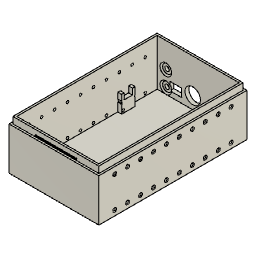
Outer Case Bottom v69 (Autodesk Fusion 360 design; units mm, degrees)
Autodesk Fusion 360 part; units mm, degrees
sketch "Sketch1" plane through (0, 0, 0) normal (0, 0, 1) x (1, 0, 0)
  line L0 (0, 0) -> (0, 12)
  line L1 (0, 12) -> (-3, 12)
  line L2 (-3, 12) -> (-3, 17)
  line L3 (-3, 17) -> (0, 17)
  line L4 (0, 17) -> (0, 79)
  line L5 (0, 79) -> (-3, 79)
  line L6 (-3, 79) -> (-3, 84)
  line L7 (-3, 84) -> (0, 84)
  line L8 (0, 84) -> (0, 96)
  line L9 (0, 96) -> (56, 96)
  line L10 (56, 96) -> (56, 84)
  line L11 (56, 84) -> (59, 84)
  line L12 (59, 84) -> (59, 79)
  line L13 (59, 79) -> (56, 79)
  line L14 (56, 79) -> (56, 17)
  line L15 (56, 17) -> (59, 17)
  line L16 (59, 17) -> (59, 12)
  line L17 (59, 12) -> (56, 12)
  line L18 (56, 12) -> (56, 0)
  line L19 (56, 0) -> (0, 0)
  line L20 (-0.7, -0.7) -> (-0.7, 11.3)
  line L21 (-0.7, 11.3) -> (-3.7, 11.3)
  line L22 (-3.7, 11.3) -> (-3.7, 17.7)
  line L23 (-3.7, 17.7) -> (-0.7, 17.7)
  line L24 (-0.7, 17.7) -> (-0.7, 78.3)
  line L25 (-0.7, 78.3) -> (-3.7, 78.3)
  line L26 (-3.7, 78.3) -> (-3.7, 84.7)
  line L27 (-3.7, 84.7) -> (-0.7, 84.7)
  line L28 (-0.7, 84.7) -> (-0.7, 96.7)
  line L29 (-0.7, 96.7) -> (56.7, 96.7)
  line L30 (56.7, 96.7) -> (56.7, 84.7)
  line L31 (56.7, 84.7) -> (59.7, 84.7)
  line L32 (59.7, 84.7) -> (59.7, 78.3)
  line L33 (59.7, 78.3) -> (56.7, 78.3)
  line L34 (56.7, 78.3) -> (56.7, 17.7)
  line L35 (56.7, 17.7) -> (59.7, 17.7)
  line L36 (59.7, 17.7) -> (59.7, 11.3)
  line L37 (59.7, 11.3) -> (56.7, 11.3)
  line L38 (56.7, 11.3) -> (56.7, -0.7)
  line L39 (56.7, -0.7) -> (-0.7, -0.7)
  line L40 (-3.7, 106.7) -> (59.7, 106.7)
  line L41 (59.7, 106.7) -> (59.7, -1.7)
  line L42 (59.7, -1.7) -> (-3.7, -1.7)
  line L43 (-3.7, -1.7) -> (-3.7, 106.7)
  line L44 (62.7, -4.7) -> (-6.7, -4.7)
  line L45 (-6.7, -4.7) -> (-6.7, 109.7)
  line L46 (-6.7, 109.7) -> (62.7, 109.7)
  line L47 (62.7, 109.7) -> (62.7, -4.7)
  line L48 (-3.7, 86.7) -> (-0.7, 86.7)
  line L49 (-0.7, 86.7) -> (-0.7, 76.3)
  line L50 (-0.7, 76.3) -> (-3.7, 76.3)
  line L51 (-3.7, 76.3) -> (-3.7, 86.7)
  line L52 (-3.7, 19.7) -> (-0.7, 19.7)
  line L53 (-0.7, 19.7) -> (-0.7, 9.3)
  line L54 (-0.7, 9.3) -> (-3.7, 9.3)
  line L55 (-3.7, 9.3) -> (-3.7, 19.7)
  line L56 (59.7, 19.7) -> (56.7, 19.7)
  line L57 (56.7, 19.7) -> (56.7, 9.3)
  line L58 (56.7, 9.3) -> (59.7, 9.3)
  line L59 (59.7, 9.3) -> (59.7, 19.7)
  line L60 (59.7, 86.7) -> (56.7, 86.7)
  line L61 (56.7, 86.7) -> (56.7, 76.3)
  line L62 (56.7, 76.3) -> (59.7, 76.3)
  line L63 (59.7, 76.3) -> (59.7, 86.7)
  dimension "d1" = 56
  dimension "d2" = 5
  dimension "d3" = 12
  dimension "d4" = 5
  dimension "d5" = 12
  dimension "d6" = 3
  dimension "d7" = 3
  dimension "d8" = -0.7
  dimension "d9" = -3
  dimension "d10" = 10
  dimension "d11" = 1
  dimension "d12" = 2
  dimension "d13" = 2
  dimension "d14" = 2
  dimension "d15" = 2
  dimension "d16" = 2
  dimension "d17" = 2
  dimension "d18" = 2
  dimension "d19" = 2
  dimension "d28" = 96
  constraint coincident L0.start L19.end
  constraint vertical L0
  constraint perpendicular L0 L1
  constraint perpendicular L1 L2
  constraint perpendicular L2 L3
  constraint perpendicular L3 L4
  constraint perpendicular L2 L5
  constraint perpendicular L5 L6
  constraint perpendicular L2 L7
  constraint perpendicular L7 L8
  constraint perpendicular L8 L9
  constraint perpendicular L9 L10
  constraint perpendicular L8 L11
  constraint perpendicular L11 L12
  constraint perpendicular L12 L13
  constraint perpendicular L13 L14
  constraint perpendicular L14 L15
  constraint perpendicular L15 L16
  constraint perpendicular L16 L17
  constraint perpendicular L17 L18
  constraint perpendicular L0 L19
  constraint collinear L4 L8
  constraint collinear L0 L4
  constraint collinear L10 L14
  constraint horizontal L6.end L11.end
  constraint horizontal L5.end L12.end
  constraint horizontal L2.end L15.end
  constraint horizontal L1.end L16.end
  constraint vertical L2.end L6.end
  constraint vertical L11.end L15.end
  constraint horizontal L40
  constraint vertical L41
  constraint horizontal L42
  constraint vertical L43
  constraint horizontal L48
  constraint vertical L49
  constraint horizontal L50
  constraint vertical L51
  constraint coincident L24 L49.end
  constraint coincident L43 L48.start
  constraint horizontal L52
  constraint vertical L53
  constraint horizontal L54
  constraint vertical L55
  constraint coincident L20 L53.end
  constraint coincident L43 L52.start
  constraint horizontal L56
  constraint vertical L57
  constraint horizontal L58
  constraint vertical L59
  constraint coincident L38 L57.end
  constraint coincident L41 L56.start
  constraint horizontal L60
  constraint vertical L61
  constraint horizontal L62
  constraint vertical L63
  constraint coincident L34 L61.end
  constraint coincident L41 L60.start
  constraint vertical L14.end L17.end
  measures "d1" distance of L8.end L9.end
  measures "d2" distance of L5.end L6.end
  measures "d3" distance of L7 L9
  measures "d4" distance of L1.end L2.end
  measures "d5" distance of L1 L19
  measures "d6" distance of L6.end L7.end
  measures "d7" distance of L10.end L11.end
  measures "d10" distance of L29 L40
  measures "d11" distance of L39 L42
  measures "d12" distance of L27 L48
  measures "d13" distance of L25 L50
  measures "d14" distance of L23 L52
  measures "d15" distance of L21 L54
  measures "d16" distance of L35 L56
  measures "d17" distance of L37 L58
  measures "d18" distance of L31 L60
  measures "d19" distance of L33 L62
  measures "d28" distance of L9 L19
extrude "Extrude4" add sketch "Sketch1" along normal blind 10.6 contours L1 L2 L3 L21 L22 L23 L43 L53 L55 | L1 L2 L3 L53 | L15 L16 L17 L57 | L15 L16 L17 L35 L36 L37 L41 L57 L59 | L5 L6 L7 L25 L26 L27 L43 L49 L51 | L5 L6 L7 L49 | L11 L12 L13 L61 | L11 L12 L13 L31 L32 L33 L41 L61 L63 makes body 1 at (56.7, 82.5667, 3.5333) makes body 2 at (59.7, 13.4333, 7.0667) makes body 3 at (-0.7, 82.5667, 3.5333) makes body 4 at (-0.7, 15.5667, 3.5333)
extrude "Extrude3" add sketch "Sketch1" along normal blind 15.2 contours L20 L21 L43 L53 L54 L55 | L23 L24 L43 L52 L53 L55 | L37 L38 L41 L57 L58 L59 | L34 L35 L41 L56 L57 L59 | L24 L25 L43 L49 L50 L51 | L33 L34 L41 L61 L62 L63 | L27 L28 L43 L48 L49 L51 | L30 L31 L41 L60 L61 L63 bodies 1 2 3 4
extrude "Extrude2" add sketch "Sketch1" along normal blind 33 bodies 1 2 3 4
extrude "Extrude1" add sketch "Sketch1" along normal blind 2 contours L0 L1 L17 L18 L19 L20 L38 L39 L53 L57 | L0 L1 L3 L4 L5 L7 L8 L9 L10 L11 L13 L14 L15 L17 L18 L19 L49 L53 L57 L61 | L1 L2 L3 L21 L22 L23 L43 L53 L55 | L1 L2 L3 L53 | L3 L4 L5 L24 L49 L53 | L20 L21 L43 L53 L54 L55 | L15 L16 L17 L57 | L15 L16 L17 L35 L36 L37 L41 L57 L59 | L23 L24 L43 L52 L53 L55 | L20 L38 L39 L41 L42 L43 L54 L58 | L13 L14 L15 L34 L57 L61 | L37 L38 L41 L57 L58 L59 | L24 L43 L50 L52 | L34 L35 L41 L56 L57 L59 | L5 L6 L7 L25 L26 L27 L43 L49 L51 | L5 L6 L7 L49 | L24 L25 L43 L49 L50 L51 | L34 L41 L56 L62 | L7 L8 L9 L10 L11 L28 L29 L30 L49 L61 | L11 L12 L13 L61 | L11 L12 L13 L31 L32 L33 L41 L61 L63 | L33 L34 L41 L61 L62 L63 | L27 L28 L43 L48 L49 L51 | L28 L29 L30 L40 L41 L43 L48 L60 | L30 L31 L41 L60 L61 L63 | L44 L45 L46 L47 bodies 1
sketch "Sketch2" plane through (0, 0, 33) normal (0, 0, 1) x (-1, 0, 0)
  line L0 (-62.7, -109.7) -> (6.7, -109.7)
  line L1 (6.7, -109.7) -> (6.7, 4.7)
  line L2 (6.7, 4.7) -> (-62.7, 4.7)
  line L3 (-62.7, 4.7) -> (-62.7, -109.7)
  line L4 (-59.7, -106.7) -> (-59.7, 1.7)
  line L5 (-59.7, 1.7) -> (3.7, 1.7)
  line L6 (3.7, 1.7) -> (3.7, -106.7)
  line L7 (3.7, -106.7) -> (-59.7, -106.7)
  line L8 (-61.2, 3.2) -> (-61.2, -108.2)
  line L9 (-61.2, -108.2) -> (5.2, -108.2)
  line L10 (5.2, -108.2) -> (5.2, 3.2)
  line L11 (5.2, 3.2) -> (-61.2, 3.2)
  line L12 (3.7, -117.1) -> (3.7, -106.7)
  line L13 (-59.7, -19.7) -> (-59.7, -9.3)
  line L14 (3.7, -86.7) -> (3.7, -76.3)
  line L15 (-59.7, -86.7) -> (-59.7, -76.3)
  dimension "d29" = -1.5
  constraint coincident L6.end L7.start
extrude "Extrude5" add sketch "Sketch2" along normal blind 5 contours L8 L9 L10 L11 bodies 1
sketch "Sketch3" plane through (0, 106.7, 0) normal (0, -1, 0) x (1, 0, 0)
  line L0 (-3.7, 2) -> (59.7, 2)
  line L1 (59.7, 2) -> (59.7, 38)
  line L2 (59.7, 38) -> (-3.7, 38)
  line L3 (-3.7, 38) -> (-3.7, 2)
  circle A0 centre (53, 6.5) radius 1.7
  circle A1 centre (3, 6.5) radius 1.7
  circle A2 centre (53, 18.5) radius 1.7
  circle A3 centre (3, 18.5) radius 1.7
  line L4 (36, 12.3) -> (47.3, 12.3)
  line L5 (47.3, 12.3) -> (47.3, 6.4)
  line L6 (47.3, 6.4) -> (36, 6.4)
  line L7 (36, 6.4) -> (36, 12.3)
  line L8 (6.2, 5.9) -> (15.1, 5.9)
  line L9 (15.1, 5.9) -> (15.1, 12.2)
  line L10 (15.1, 12.2) -> (6.2, 12.2)
  line L11 (6.2, 12.2) -> (6.2, 5.9)
  line L12 (36, 12.3) -> (33, 12.3)
  line L13 (33, 12.3) -> (33, 14.3)
  line L14 (33, 14.3) -> (36, 14.3)
  line L15 (36, 14.3) -> (36, 12.3)
  line L16 (36, 6.4) -> (33, 6.4)
  line L17 (33, 6.4) -> (33, 4.4)
  line L18 (33, 4.4) -> (36, 4.4)
  line L19 (36, 4.4) -> (36, 6.4)
  line L20 (47.3, 12.3) -> (50.3, 12.3)
  line L21 (50.3, 12.3) -> (50.3, 14.3)
  line L22 (50.3, 14.3) -> (47.3, 14.3)
  line L23 (47.3, 14.3) -> (47.3, 12.3)
  line L24 (47.3, 6.4) -> (50.3, 6.4)
  line L25 (50.3, 6.4) -> (50.3, 4.4)
  line L26 (50.3, 4.4) -> (47.3, 4.4)
  line L27 (47.3, 4.4) -> (47.3, 6.4)
  circle A4 centre (3, 18.5) radius 3.5
  circle A5 centre (3, 6.5) radius 3.5
  circle A6 centre (53, 18.5) radius 3.5
  circle A7 centre (53, 6.5) radius 3.5
  dimension "d32" = 3.4
  dimension "d35" = -50
  dimension "d36" = 12
  dimension "d37" = 4.5
  dimension "d38" = 6.7
  dimension "d41" = 50
  dimension "d42" = 63.4
  dimension "d43" = 12.4
  dimension "d45" = 5.9
  dimension "d46" = 11.3
  dimension "d47" = 8.9
  dimension "d48" = 6.3
  dimension "d49" = 3.9
  dimension "d51" = 3
  dimension "d52" = 2
  dimension "d53" = 3
  dimension "d54" = 2
  dimension "d55" = 3
  dimension "d56" = 2
  dimension "d57" = 3
  dimension "d58" = 2
  dimension "d74" = 4.4
  dimension "d75" = 7
  dimension "d76" = 7
  dimension "d77" = 7
  dimension "d78" = 7
  dimension "d113" = 9.9
  constraint horizontal L4
  constraint vertical L5
  constraint horizontal L6
  constraint vertical L7
  constraint horizontal L8
  constraint vertical L9
  constraint horizontal L10
  constraint vertical L11
  constraint horizontal L12
  constraint vertical L13
  constraint horizontal L14
  constraint vertical L15
  constraint horizontal L16
  constraint vertical L17
  constraint horizontal L18
  constraint vertical L19
  constraint horizontal L20
  constraint vertical L21
  constraint horizontal L22
  constraint vertical L23
  constraint horizontal L24
  constraint vertical L25
  constraint horizontal L26
  constraint vertical L27
  constraint concentric A3 A4
  constraint concentric A1 A5
  constraint concentric A2 A6
  constraint concentric A0 A7
  measures "d32" diameter of A0
  measures "d37" distance of L0 A0.centre
  measures "d38" distance of L1 A0.centre
  measures "d41" distance of A2.centre A3.centre
  measures "d42" distance of L1.end L2.end
  measures "d43" distance of L1 L5
  measures "d45" distance of L4.start L6.end
  measures "d46" distance of L4.start L4.end
  measures "d47" distance of L8.start L8.end
  measures "d48" distance of L8.start L10.end
  measures "d49" distance of L0 L8
  measures "d51" distance of L4.start L12.end
  measures "d52" distance of L4.start L14.end
  measures "d53" distance of L6.end L16.end
  measures "d54" distance of L6.end L18.end
  measures "d55" distance of L4.end L20.end
  measures "d56" distance of L4.end L22.end
  measures "d57" distance of L5.end L24.end
  measures "d58" distance of L5.end L26.end
  measures "d74" distance of L0 L6
  measures "d75" diameter of A4
  measures "d76" diameter of A5
  measures "d77" diameter of A6
  measures "d78" diameter of A7
  measures "d113" distance of L3 L11
extrude "Extrude9" cut sketch "Sketch3" against normal blind 1 contours L24 L25 L26 A7 | L24 L25 L26 A7 | L8 L11 A5 | L8 L11 A5 | A4 | A6 bodies 1
extrude "Extrude6" cut sketch "Sketch3" against normal blind 4 contours A0 | A1 | A2 | A3 | L4 L5 L6 L7 | L8 L11 A5 | L8 L9 L10 L11 A5 picked at (6.2552, 7.0928) bodies 1
sketch "Sketch6" plane through (0, 0, 2) normal (0, 0, 1) x (-1, 0, 0)
  line L0 (-59.7, -86.7) -> (-59.7, -106.7)
  line L1 (-59.7, -106.7) -> (3.7, -106.7)
  line L2 (3.7, -106.7) -> (3.7, -86.7)
  line L3 (3.7, -86.7) -> (0.7, -86.7)
  line L4 (0.7, -86.7) -> (0.7, -76.3)
  line L5 (0.7, -76.3) -> (3.7, -76.3)
  line L6 (3.7, -76.3) -> (3.7, -19.7)
  line L7 (3.7, -19.7) -> (0.7, -19.7)
  line L8 (0.7, -19.7) -> (0.7, -9.3)
  line L9 (0.7, -9.3) -> (3.7, -9.3)
  line L10 (3.7, -9.3) -> (3.7, 1.7)
  line L11 (3.7, 1.7) -> (-59.7, 1.7)
  line L12 (-59.7, 1.7) -> (-59.7, -9.3)
  line L13 (-59.7, -9.3) -> (-56.7, -9.3)
  line L14 (-56.7, -9.3) -> (-56.7, -19.7)
  line L15 (-56.7, -19.7) -> (-59.7, -19.7)
  line L16 (-59.7, -19.7) -> (-59.7, -76.3)
  line L17 (-59.7, -76.3) -> (-56.7, -76.3)
  line L18 (-56.7, -76.3) -> (-56.7, -86.7)
  line L19 (-56.7, -86.7) -> (-59.7, -86.7)
  line L20 (-17.3, -15.8) -> (-27.3, -15.8)
  line L21 (-27.3, -15.8) -> (-27.3, -5.8)
  line L22 (-27.3, -5.8) -> (-17.3, -5.8)
  line L23 (-17.3, -5.8) -> (-17.3, -15.8)
  line L24 (-30.3, -18.8) -> (-14.3, -18.8)
  line L25 (-14.3, -18.8) -> (-14.3, -2.8)
  line L26 (-14.3, -2.8) -> (-30.3, -2.8)
  line L27 (-30.3, -2.8) -> (-30.3, -18.8)
  dimension "d87" = 10
  dimension "d88" = 10
  dimension "d89" = 7.5
  dimension "d96" = 21
  dimension "d97" = 16
  dimension "d98" = 16
  dimension "d99" = 3
  dimension "d100" = 3
  constraint horizontal L20
  constraint vertical L21
  constraint horizontal L22
  constraint vertical L23
  constraint horizontal L24
  constraint vertical L25
  constraint horizontal L26
  constraint vertical L27
  measures "d87" distance of L20.start L20.end
  measures "d88" distance of L20.start L22.end
  measures "d89" distance of L11 L22
  measures "d96" distance of L10 L23
  measures "d97" distance of L24.start L24.end
  measures "d98" distance of L24.start L26.end
  measures "d99" distance of L20 L24
  measures "d100" distance of L21 L27
extrude "Extrude12" cut sketch "Sketch6" against normal blind 1 contours L24 L25 L26 L27 bodies 1
extrude "Extrude11" cut sketch "Sketch6" against normal blind 3 contours L20 L21 L22 L23 bodies 1
chamfer "Chamfer3" distance 0.5 angle 45 4 edges at (22.3, 5.8, 0) (17.3, 10.8, 0) (22.3, 15.8, 0) (27.3, 10.8, 0) measured on face at (27.7667, 78.4, 0) measured on face at (27.7667, 78.4, 0) measured on face at (27.7667, 78.4, 0) measured on face at (27.7667, 78.4, 0) on bodies 1
sketch "Sketch7" plane through (0, -3.2, 0) normal (0, -1, 0) x (1, 0, 0)
  line L0 (-5.2, 33) -> (61.2, 33)
  line L1 (61.2, 33) -> (61.2, 38)
  line L2 (61.2, 38) -> (-5.2, 38)
  line L3 (-5.2, 38) -> (-5.2, 33)
  line L4 (12, 33) -> (44, 33)
  line L5 (44, 33) -> (44, 34.5)
  line L6 (44, 34.5) -> (12, 34.5)
  line L7 (12, 34.5) -> (12, 33)
  dimension "d103" = 32
  dimension "d104" = 1.5
  dimension "d105" = 66.4
  dimension "d106" = 17.2
  constraint horizontal L4
  constraint vertical L5
  constraint horizontal L6
  constraint vertical L7
  constraint coincident L0 L4.start
  measures "d103" distance of L4.start L4.end
  measures "d104" distance of L4.start L6.end
  measures "d105" distance of L1.end L2.end
  measures "d106" distance of L1 L5
revolve "Revolve1" cut sketch "Sketch7" angle 25 about axis through (44, -3.2, 34.5) along (1, 0, 0) contours L0 L4 L5 L6 L7 bodies 1
sketch "Sketch8" plane through (0, 108.2, 0) normal (0, 1, 0) x (-1, 0, 0)
  line L0 (-61.2, 33) -> (5.2, 33)
  line L1 (5.2, 33) -> (5.2, 38)
  line L2 (5.2, 38) -> (-61.2, 38)
  line L3 (-61.2, 38) -> (-61.2, 33)
  line L4 (-44, 33) -> (-12, 33)
  line L5 (-12, 33) -> (-12, 34.5)
  line L6 (-12, 34.5) -> (-44, 34.5)
  line L7 (-44, 34.5) -> (-44, 33)
  dimension "d108" = 32
  dimension "d109" = 1.5
  dimension "d110" = 66.4
  dimension "d111" = 17.2
  constraint horizontal L4
  constraint vertical L5
  constraint horizontal L6
  constraint vertical L7
  constraint coincident L0 L4.start
  measures "d108" distance of L4.start L4.end
  measures "d109" distance of L4.start L6.end
  measures "d110" distance of L1.end L2.end
  measures "d111" distance of L1 L5
revolve "Revolve2" cut sketch "Sketch8" angle 25 about axis through (12, 108.2, 34.5) along (-1, 0, 0) contours L0 L4 L5 L6 L7 bodies 1
sketch "Sketch9" plane through (0, 109.7, 0) normal (0, 1, 0) x (-1, 0, 0)
  circle A0 centre (-53, 18.5) radius 1.7
  circle A1 centre (-3, 18.5) radius 1.7
  line L0 (-47.3, 6.4) -> (-47.3, 12.3)
  line L1 (-47.3, 12.3) -> (-36, 12.3)
  line L2 (-36, 12.3) -> (-36, 6.4)
  line L3 (-36, 6.4) -> (-47.3, 6.4)
  circle A2 centre (-53, 6.5) radius 1.7
  circle A3 centre (-3, 6.5) radius 1.7
  line L4 (-6.2, 5.9) -> (-15.1, 5.9)
  line L5 (-15.1, 5.9) -> (-15.1, 12.2)
  line L6 (-15.1, 12.2) -> (-6.2, 12.2)
  line L7 (-6.2, 12.2) -> (-6.2, 5.9)
  line L8 (6.7, 0) -> (6.7, 33)
  line L9 (6.7, 33) -> (-62.7, 33)
  line L10 (-62.7, 33) -> (-62.7, 0)
  line L11 (-62.7, 0) -> (6.7, 0)
  circle A4 centre (-23.8, 11.38) radius 6
  dimension "d114" = 12
  dimension "d115" = 11.38
  dimension "d116" = 30.5
  measures "d114" diameter of A4
  measures "d115" distance of L11 A4.centre
  measures "d116" distance of L8 A4.centre
extrude "Extrude13" cut sketch "Sketch9" against normal blind 4 contours A4 bodies 1
chamfer "Chamfer4" distance 1 angle 45 4 edges at (-0.2631, 106.7, 19.7657) (-0.4738, 106.7, 6.0727) (49.7369, 106.7, 19.7657) (49.7369, 106.7, 7.7657) on bodies 1
sketch "Sketch11" plane through (0, 9.3, 0) normal (0, -1, 0) x (1, 0, 0)
  line L0 (-3.7, 2) -> (-0.7, 2)
  line L1 (-0.7, 2) -> (-0.7, 15.2)
  line L2 (-0.7, 15.2) -> (-3.7, 15.2)
  line L3 (-3.7, 15.2) -> (-3.7, 2)
  line L4 (-0.7, 10.6) -> (-3.7, 10.6)
  line L5 (-3.7, 10.6) -> (-3.7, 8.6)
  line L6 (-3.7, 8.6) -> (-0.7, 8.6)
  line L7 (-0.7, 8.6) -> (-0.7, 10.6)
  line L8 (56.7, 10.6) -> (59.7, 10.6)
  line L9 (59.7, 10.6) -> (59.7, 8.6)
  line L10 (59.7, 8.6) -> (56.7, 8.6)
  line L11 (56.7, 8.6) -> (56.7, 10.6)
  line L12 (56.7, 2) -> (56.7, 15.2)
  line L13 (59.7, 15.2) -> (59.7, 2)
  line L14 (56.7, 15.2) -> (59.7, 15.2)
  dimension "d120" = 2
  dimension "d121" = 4.6
  dimension "d123" = 2
  dimension "d124" = 4.6
  constraint horizontal L4
  constraint vertical L5
  constraint horizontal L6
  constraint vertical L7
  constraint coincident L1 L4.start
  constraint horizontal L8
  constraint vertical L9
  constraint horizontal L10
  constraint vertical L11
  constraint coincident L8.start L12
  constraint coincident L8.end L13
  measures "d120" distance of L4.start L6.end
  measures "d121" distance of L2 L4
  measures "d123" distance of L8.start L10.end
  measures "d124" distance of L8.start L12.end
revolve "Revolve3" cut sketch "Sketch11" angle 15 about axis through (-0.7, 9.3, 10.6) along (1, 0, 0) contours L1 L3 L4 L5 L6 L7 | L8 L9 L10 L11 L12 L13 bodies 1
sketch "Sketch12" plane through (0, 76.3, 0) normal (0, -1, 0) x (1, 0, 0)
  line L0 (-3.7, 2) -> (-0.7, 2)
  line L1 (-0.7, 2) -> (-0.7, 15.2)
  line L2 (-0.7, 15.2) -> (-3.7, 15.2)
  line L3 (-3.7, 15.2) -> (-3.7, 2)
  line L4 (-0.7, 10.6) -> (-3.7, 10.6)
  line L5 (-3.7, 10.6) -> (-3.7, 8.6)
  line L6 (-3.7, 8.6) -> (-0.7, 8.6)
  line L7 (-0.7, 8.6) -> (-0.7, 10.6)
  line L8 (59.7, 8.6) -> (56.7, 8.6)
  line L9 (56.7, 8.6) -> (56.7, 10.6)
  line L10 (56.7, 10.6) -> (59.7, 10.6)
  line L11 (59.7, 10.6) -> (59.7, 8.6)
  line L12 (56.7, 15.2) -> (59.7, 15.2)
  line L13 (56.7, 2) -> (56.7, 15.2)
  dimension "d128" = 2
  dimension "d129" = 4.6
  dimension "d130" = 3
  dimension "d131" = 2
  dimension "d132" = 4.6
  constraint horizontal L4
  constraint vertical L5
  constraint horizontal L6
  constraint vertical L7
  constraint coincident L1 L4.start
  constraint horizontal L8
  constraint vertical L9
  constraint horizontal L10
  constraint vertical L11
  constraint coincident L9.end L13
  measures "d128" distance of L4.start L6.end
  measures "d129" distance of L2 L4
  measures "d130" distance of L8.start L8.end
  measures "d131" distance of L8.start L10.end
  measures "d132" distance of L10 L12
revolve "Revolve4" cut sketch "Sketch12" angle 15 about axis through (56.7, 76.3, 10.6) along (1, 0, 0) contours L1 L3 L4 L5 L6 L7 | L8 L9 L10 L11 L13 bodies 1
sketch "Sketch13" plane through (0, 86.7, 0) normal (0, 1, 0) x (-1, 0, 0)
  line L0 (-59.7, 2) -> (-56.7, 2)
  line L1 (-56.7, 2) -> (-56.7, 15.2)
  line L2 (-56.7, 15.2) -> (-59.7, 15.2)
  line L3 (-59.7, 15.2) -> (-59.7, 2)
  line L4 (-56.7, 10.6) -> (-59.7, 10.6)
  line L5 (-59.7, 10.6) -> (-59.7, 8.6)
  line L6 (-59.7, 8.6) -> (-56.7, 8.6)
  line L7 (-56.7, 8.6) -> (-56.7, 10.6)
  line L8 (3.7, 10.6) -> (0.7, 10.6)
  line L9 (0.7, 10.6) -> (0.7, 8.6)
  line L10 (0.7, 8.6) -> (3.7, 8.6)
  line L11 (3.7, 8.6) -> (3.7, 10.6)
  line L12 (0.7, 2) -> (0.7, 15.2)
  point P0 (0.7, 15.2)
  dimension "d134" = 2
  dimension "d135" = 4.6
  dimension "d136" = 3
  dimension "d137" = 2
  dimension "d138" = 4.6
  constraint horizontal L4
  constraint vertical L5
  constraint horizontal L6
  constraint vertical L7
  constraint coincident L3 L5.end
  constraint coincident L1 L4.start
  constraint horizontal L8
  constraint vertical L9
  constraint horizontal L10
  constraint vertical L11
  constraint coincident L8.end L12
  measures "d134" distance of L4.start L6.end
  measures "d135" distance of L2 L4
  measures "d136" distance of L8.start L8.end
  measures "d137" distance of L8.start L10.end
  measures "d138" distance of L8 P0
revolve "Revolve5" cut sketch "Sketch13" angle 15 about axis through (56.7, 86.7, 10.6) along (-1, 0, 0) contours L1 L3 L4 L5 L6 L7 | L8 L9 L10 L11 L12 bodies 1
sketch "Sketch14" plane through (0, 19.7, 0) normal (0, 1, 0) x (-1, 0, 0)
  line L0 (-59.7, 2) -> (-56.7, 2)
  line L1 (-56.7, 2) -> (-56.7, 15.2)
  line L2 (-56.7, 15.2) -> (-59.7, 15.2)
  line L3 (-59.7, 15.2) -> (-59.7, 2)
  line L4 (-56.7, 10.6) -> (-59.6993, 10.6)
  line L5 (-59.6993, 10.6) -> (-59.6993, 8.6)
  line L6 (-59.6993, 8.6) -> (-56.7, 8.6)
  line L7 (-56.7, 8.6) -> (-56.7, 10.6)
  line L8 (3.7, 10.6) -> (0.7, 10.6)
  line L9 (0.7, 10.6) -> (0.7, 8.6)
  line L10 (0.7, 8.6) -> (3.7, 8.6)
  line L11 (3.7, 8.6) -> (3.7, 10.6)
  line L12 (0.7, 2) -> (0.7, 15.2)
  point P0 (0.7, 15.2)
  dimension "d140" = 2
  dimension "d141" = 4.6
  dimension "d142" = 3
  dimension "d143" = 2
  dimension "d144" = 4.6
  constraint horizontal L4
  constraint vertical L5
  constraint horizontal L6
  constraint vertical L7
  constraint coincident L1 L4.start
  constraint horizontal L8
  constraint vertical L9
  constraint horizontal L10
  constraint vertical L11
  constraint coincident L8.end L12
  measures "d140" distance of L4.start L6.end
  measures "d141" distance of L2 L4
  measures "d142" distance of L8.start L8.end
  measures "d143" distance of L8.start L10.end
  measures "d144" distance of L8 P0
revolve "Revolve6" cut sketch "Sketch14" angle 15 about axis through (56.7, 19.7, 10.6) along (-1, 0, 0) contours L1 L3 L4 L5 L6 L7 | L8 L9 L10 L11 L12 bodies 1
sketch "Sketch16" plane through (62.7, 0, 0) normal (1, 0, 0) x (0, 1, 0)
  line L0 (109.7, 0) -> (109.7, 33)
  line L1 (109.7, 33) -> (-4.7, 33)
  line L2 (-4.7, 33) -> (-4.7, 0)
  line L3 (-4.7, 0) -> (109.7, 0)
  circle A0 centre (7.5, 4) radius 1
  circle A1 centre (7.5, 28) radius 1
  dimension "d146" = 2
  dimension "d147" = 4
  dimension "d148" = 12.2
  dimension "d166" = 2
  dimension "d167" = 5
  measures "d146" diameter of A0
  measures "d147" distance of L3 A0.centre
  measures "d148" distance of L2 A0.centre
  measures "d166" diameter of A1
  measures "d167" distance of L1 A1.centre
extrude "Extrude14" cut sketch "Sketch16" against normal blind 10 contours A0 | A1 bodies 1
chamfer "Chamfer5" distance 0.5 angle 45 1 edges at (62.7, 6.5677, 4.3616) on bodies 1
chamfer "Chamfer7" distance 0.5 angle 45 1 edges at (62.7, 6.5677, 28.3616) on bodies 1
pattern_linear "R-Pattern3" count 10 spacing 10 along (0, 1, 0) of "Extrude14", "Chamfer5", "Chamfer7"
sketch "Sketch17" plane through (-6.7, 0, 0) normal (-1, 0, 0) x (0, -1, 0)
  line L0 (4.7, 0) -> (4.7, 33)
  line L1 (4.7, 33) -> (-109.7, 33)
  line L2 (-109.7, 33) -> (-109.7, 0)
  line L3 (-109.7, 0) -> (4.7, 0)
  circle A0 centre (-97.5, 4) radius 1
  circle A1 centre (-97.5, 28) radius 1
  dimension "d156" = 2
  dimension "d157" = 4
  dimension "d158" = 12.2
  dimension "d173" = 2
  dimension "d174" = 5
  measures "d156" diameter of A0
  measures "d157" distance of L3 A0.centre
  measures "d158" distance of L2 A0.centre
  measures "d173" diameter of A1
  measures "d174" distance of L1 A1.centre
extrude "Extrude15" cut sketch "Sketch17" against normal blind 10 contours A0 | A1 bodies 1
chamfer "Chamfer8" distance 0.5 angle 45 2 edges at (-6.7, 98.4323, 4.3616) (-6.7, 98.4323, 28.3616) on bodies 1
pattern_linear "R-Pattern4" count 10 spacing 10 along (0, -1, 0) of "Extrude15", "Chamfer8"
sketch "Sketch15" plane through (59.7, 0, 0) normal (-1, 0, 0) x (0, -1, 0)
  line L0 (-9.3, 2) -> (1.7, 2)
  line L1 (1.7, 2) -> (1.7, 38)
  line L2 (1.7, 38) -> (-106.7, 38)
  line L3 (-106.7, 38) -> (-106.7, 2)
  line L4 (-106.7, 2) -> (-86.7, 2)
  line L5 (-86.7, 4.6) -> (-86.7, 8.6)
  arc A0 (-86.7, 8.6) -> (-86.1824, 8.6681) centre (-86.7, 10.6) ccw
  line L6 (-86.1824, 8.6681) -> (-86.7, 10.6)
  line L7 (-86.7, 10.6) -> (-86.7, 15.2)
  line L8 (-86.7, 15.2) -> (-84.7, 15.2)
  line L9 (-84.7, 15.2) -> (-84.7, 10.6)
  line L10 (-84.7, 10.6) -> (-78.3, 10.6)
  line L11 (-78.3, 10.6) -> (-78.3, 15.2)
  line L12 (-78.3, 15.2) -> (-76.3, 15.2)
  line L13 (-76.3, 15.2) -> (-76.3, 10.6)
  line L14 (-76.3, 10.6) -> (-76.8176, 8.6681)
  arc A1 (-76.8176, 8.6681) -> (-76.3, 8.6) centre (-76.3, 10.6) ccw
  line L15 (-76.3, 8.6) -> (-76.3, 2)
  line L16 (-76.3, 2) -> (-19.7, 2)
  line L17 (-19.7, 2) -> (-19.7, 15.2)
  line L18 (-19.7, 15.2) -> (-17.7, 15.2)
  line L19 (-17.7, 15.2) -> (-17.7, 10.6)
  line L20 (-17.7, 10.6) -> (-11.3, 10.6)
  line L21 (-11.3, 10.6) -> (-11.3, 15.2)
  line L22 (-11.3, 15.2) -> (-9.3, 15.2)
  line L23 (-9.3, 15.2) -> (-9.3, 10.6)
  line L24 (-9.3, 10.6) -> (-9.8176, 8.6681)
  arc A2 (-9.8176, 8.6681) -> (-9.3, 8.6) centre (-9.3, 10.6) ccw
  line L25 (-9.3, 8.6) -> (-9.3, 2)
  spline S0 degree 5 poles (-88.5, 17) (-88.3083, 17.0643) (-87.874, 17.1854) (-87.0666, 17.3513) (-85.69, 17.5583) (-83.5901, 17.7891) (-81.2922, 17.9551) (-79.0071, 18.0016) (-76.9457, 17.8695) (-75.2874, 17.5101) (-74.1518, 16.8982) (-73.5635, 16.0488) (-73.4355, 15.0239) (-73.6166, 13.9078) (-73.9295, 12.7856) (-74.2104, 11.7235) (-74.3535, 10.7418) (-74.3195, 9.8256) (-74.1327, 8.9494) (-73.8786, 8.0947) (-73.709, 7.2766) (-73.8168, 6.5439) (-74.3746, 5.9499) (-75.4825, 5.5308) (-77.1137, 5.2816) (-79.1475, 5.1702) (-81.4009, 5.1501) (-83.6614, 5.1744) (-85.7176, 5.2084) (-87.3926, 5.244) (-88.573, 5.3102) (-89.2484, 5.494) (-89.5163, 5.9288) (-89.5236, 6.7287) (-89.4157, 7.923) (-89.3001, 9.427) (-89.2489, 11.0925) (-89.292, 12.7405) (-89.4136, 14.2016) (-89.5489, 15.3503) (-89.5755, 16.1497) (-89.3729, 16.5647) (-89.0241, 16.7993) (-88.6917, 16.9357) (-88.5, 17) knots 0 0 0 0 0 0 0.025 0.05 0.075 0.1 0.125 0.15 0.175 0.2 0.225 0.25 0.275 0.3 0.325 0.35 0.375 0.4 0.425 0.45 0.475 0.5 0.525 0.55 0.575 0.6 0.625 0.65 0.675 0.7 0.725 0.75 0.775 0.8 0.825 0.85 0.875 0.9 0.925 0.95 0.975 1 1 1 1 1 1
  circle A3 centre (-7.5, 4) radius 1
  circle A4 centre (-7.5, 28) radius 1
  circle A5 centre (-97.5, 4) radius 1
  circle A6 centre (-97.5, 28) radius 1
  arc A7 (-86.7, 4.6) -> (-86.7, 3.4) centre (-87.5, 4) ccw
  line L26 (-86.7, 2) -> (-86.7, 3.4)
  circle A8 centre (-17.5, 28) radius 1
  circle A9 centre (-27.5, 28) radius 1
  circle A10 centre (-27.5, 4) radius 1
  circle A11 centre (-37.5, 28) radius 1
  circle A12 centre (-37.5, 4) radius 1
  circle A13 centre (-47.5, 28) radius 1
  circle A14 centre (-47.5, 4) radius 1
  circle A15 centre (-57.5, 28) radius 1
  circle A16 centre (-57.5, 4) radius 1
  circle A17 centre (-67.5, 28) radius 1
  circle A18 centre (-67.5, 4) radius 1
  circle A19 centre (-77.5, 28) radius 1
  circle A20 centre (-87.5, 28) radius 1
  point P0 (-74.5, 17)
  point P1 (-74, 12.5)
  point P2 (-74, 8.5)
  point P3 (-74.5, 6)
  point P4 (-88.0921, 5.3)
  point P5 (-89.5, 6.5)
  point P6 (-89.5, 15)
split "Split1" [suppressed]
equation "d4 = d2"
equation "d5 = d3"
equation "d13 = d12"
equation "d14 = d12"
equation "d15 = d12"
equation "d16 = d12"
equation "d17 = d12"
equation "d18 = d12"
equation "d19 = d12"
equation "d38 = ( 63.40 mm - d41 ) / 2"
equation "d43 = 12.5 mm - 0.1 mm"
equation "d49 = 3 mm - 0.1 mm + 1 mm"
equation "d74 = 3.5 mm - 0.1 mm + 1 mm"
equation "d99 = ( d98 - d88 ) / 2"
equation "d100 = ( d97 - d87 ) / 2"
equation "d106 = ( 66.40 mm - d103 ) / 2"
equation "d111 = ( 66.40 mm - d108 ) / 2"
equation "d113 = 10 mm - 0.1 mm"
equation "d148 = ( ( 114.4 - 90 ) / 2 ) * 1 mm"
equation "d158 = ( ( 114.4 - 90 ) / 2 ) * 1 mm"
